PLATE_HV_FRONT (Autodesk Fusion 360 design; units mm, degrees)
Autodesk Fusion 360 part; units mm, degrees
sketch "Esquisse1" plane through (0, 0, 0) normal (0, 0, 1) x (1, 0, 0)
  line L0 (75, -23) -> (-75, -23)
  line L1 (-75, -23) -> (-75, 23)
  line L2 (-75, 23) -> (75, 23)
  line L3 (75, 23) -> (75, -23)
  line L4 (75, -23) -> (-75, 23) construction
  line L5 (-75, -23) -> (75, 23) construction
  line L6 (78, -20) -> (-78, -20)
  line L7 (-78, -20) -> (-78, 20)
  line L8 (-78, 20) -> (78, 20)
  line L9 (78, 20) -> (78, -20)
  line L10 (78, -20) -> (-78, 20) construction
  line L11 (-78, -20) -> (78, 20) construction
  dimension "d1" = 150
  dimension "d2" = 46
  dimension "d57" = 156
  dimension "d58" = 40
  constraint horizontal L0
  constraint perpendicular L0 L1
  constraint parallel L0 L2
  constraint parallel L1 L3
  constraint coincident L4 origin
  constraint coincident L5 origin
  constraint horizontal L6
  constraint perpendicular L6 L7
  constraint parallel L6 L8
  constraint parallel L7 L9
  constraint coincident L10 origin
  constraint coincident L11 origin
  measures "d1" distance of L1.end L2.end
  measures "d2" distance of L0.end L1.end
  measures "d57" distance of L7.end L8.end
  measures "d58" distance of L6.end L7.end
extrude "Extrusion1" add sketch "Esquisse1" along normal blind 3
sketch "Esquisse5" plane through (0, 0, 3) normal (0, 0, 1) x (-1, 0, 0)
  line L0 (-75, -23) -> (75, -23)
  line L1 (75, -23) -> (75, -20)
  line L2 (75, 23) -> (-75, 23)
  line L3 (-75, -20) -> (-75, -23)
  circle A0 centre (18.375, -5) radius 2
  circle A1 centre (-18.375, -5) radius 2
  line L4 (-78, -20) -> (-75, -20)
  line L5 (75, -20) -> (78, -20)
  line L6 (78, -20) -> (78, 20)
  line L7 (78, 20) -> (75, 20)
  line L8 (75, 20) -> (75, 23)
  line L9 (-75, 23) -> (-75, 20)
  line L10 (-75, 20) -> (-78, 20)
  line L11 (-78, 20) -> (-78, -20)
  dimension "d49" = 4
  dimension "d50" = 4
  dimension "d53" = 36.75
  dimension "d54" = 18.375
  dimension "d59" = 5
  dimension "d60" = 5
  measures "d49" diameter of A0
  measures "d50" diameter of A1
  measures "d53" distance of A0.centre A1.centre
  measures "d54" horizontal distance of origin A0.centre
  measures "d59" vertical distance of origin A0.centre
  measures "d60" vertical distance of origin A1.centre
extrude "Extrusion6" cut sketch "Esquisse5" against normal blind 3 contours A0 | A1
equation "d2 = d58 + ( 2 * 3 ) * 1 mm"
equation "d54 = d53 / 2"
equation "d60 = d59"
